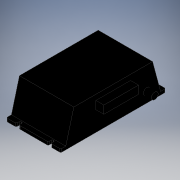
# Autodesk Inventor part: 12v_dc_to_dc
Saved by Autodesk Inventor 2017 (Build 210142000, 142)
## iProperties
Created: 2017-02-10
Part Number: 12v_dc_to_dc
Material: Generic
Document SubType Name: Modeling
Designer: michael
Density: 1 g/cm^3
Appearance: Default
Author: michael
Autodesk Inventor part; units mm, degrees
ref_plane "YZ Plane" through (0, 0, 0) normal (1, 0, 0) x (0, 1, 0)
ref_plane "XZ Plane" through (0, 0, 0) normal (0, 1, 0) x (-1, 0, 0)
ref_plane "XY Plane" through (0, 0, 0) normal (0, 0, 1) x (1, 0, 0)
sketch "Sketch1" plane through (0, 0, 0) normal (0, 1, 0) x (-1, 0, 0)
  line L0 (-51, 98.425) -> (51, 98.425)
  line L1 (51, 98.425) -> (51, -98.425)
  line L2 (51, -98.425) -> (-51, -98.425)
  line L3 (-51, -98.425) -> (-51, 98.425)
  line L4 (-51, 98.425) -> (51, -98.425) construction
  line L5 (51, 98.425) -> (-51, -98.425) construction
  point P0 (0, 0)
  dimension "d0" = 102
  dimension "d1" = 196.85
  constraints: 12 end point, 2 midpoint, 2 parallel, 1 horizontal, 1 perpendicular
  measures "d0" distance of L1.end L2.end
  measures "d1" distance of L0.end L1.end
extrude "Extrusion1" add sketch "Sketch1" along normal blind 6
sketch "Sketch2" plane through (0, 6, 0) normal (0, 1, 0) x (1, 0, 0)
  line L0 (51, -88.9) -> (-51, -88.9)
  line L1 (-51, -88.9) -> (-51, 88.9)
  line L2 (-51, 88.9) -> (51, 88.9)
  line L3 (51, 88.9) -> (51, -88.9)
  line L4 (51, -88.9) -> (-51, 88.9) construction
  line L5 (-51, -88.9) -> (51, 88.9) construction
  point P0 (0, 0)
  dimension "d4" = 102
  dimension "d5" = 177.8
  constraints: 12 end point, 2 midpoint, 2 parallel, 1 horizontal, 1 perpendicular
  measures "d4" distance of L1.end L2.end
  measures "d5" distance of L0.end L1.end
extrude "Extrusion2" add sketch "Sketch2" along normal blind 56
draft "FaceDraft1" angle 15 pull direction (0, 1, 0) faces at (17, 24.6667, 88.9) fixed edges at (0, 6, 88.9)
draft "FaceDraft2" angle 15 pull direction (0, 1, 0) faces at (-17, 24.6667, -88.9) fixed edges at (0, 6, -88.9)
sketch "Sketch3" plane through (0, 0, 0) normal (0, -1, 0) x (1, 0, 0)
  line L0 (32.4713, 98.425) -> (27.4713, 98.425)
  line L1 (27.4713, 98.425) -> (27.4713, 90.925)
  line L2 (27.4713, 90.925) -> (32.4713, 90.925)
  line L3 (32.4713, 90.925) -> (32.4713, 98.425)
  line L4 (32.4713, 98.425) -> (27.4713, 90.925) construction
  line L5 (27.4713, 98.425) -> (32.4713, 90.925) construction
  line L6 (51, -98.425) -> (51, 98.425) projected
  line L7 (-51, 98.425) -> (51, 98.425) projected
  line L8 (-27.4727, 90.925) -> (-32.4727, 90.925)
  line L9 (-32.4727, 90.925) -> (-32.4727, 98.425)
  line L10 (-32.4727, 98.425) -> (-27.4727, 98.425)
  line L11 (-27.4727, 98.425) -> (-27.4727, 90.925)
  line L12 (-27.4727, 90.925) -> (-32.4727, 98.425) construction
  line L13 (-32.4727, 90.925) -> (-27.4727, 98.425) construction
  line L14 (-51, 98.425) -> (-51, -98.425) projected
  line L15 (51, 0) -> (-51, 0)
  line L16 (-51, -73.8948) -> (-51, 73.8948) projected
  line L17 (32.4713, -98.425) -> (27.4713, -98.425)
  line L18 (27.4713, -98.425) -> (27.4713, -90.925)
  line L19 (27.4713, -90.925) -> (32.4713, -90.925)
  line L20 (32.4713, -90.925) -> (32.4713, -98.425)
  line L21 (-27.4727, -90.925) -> (-32.4727, -90.925)
  line L22 (-32.4727, -90.925) -> (-32.4727, -98.425)
  line L23 (-32.4727, -98.425) -> (-27.4727, -98.425)
  line L24 (-27.4727, -98.425) -> (-27.4727, -90.925)
  point P0 (0, 0)
  point P1 (29.9713, 94.675)
  point P2 (-29.9727, 94.675)
  point P3 (29.9713, -94.675)
  dimension "d10" = 5
  dimension "d11" = 7.5
  dimension "d12" = 21.0287
  dimension "d13" = 7.5
  dimension "d14" = 5
  dimension "d16" = 59.944
  dimension "d17" = 0
  constraints: 42 end point, 9 symmetric about line, 6 midpoint, 4 parallel, 2 horizontal, 2 perpendicular, 1 point on line
  measures "d10" distance of L2.end L1.end
  measures "d11" distance of L1.end L0.end
  measures "d12" distance from line of point (29.971, 94.675) L6
  measures "d13" distance between parallel lines of L8 L7
  measures "d14" distance between parallel lines of L9 L11
  measures "d16" distance of point (-29.973, 94.675) point (29.971, 94.675)
  measures "d17" distance between parallel lines of L7 L0
extrude "Extrusion3" cut sketch "Sketch3" against normal blind 56 contours L3 L2 L1 L0 | L11 L8 L9 L7 | L17 L18 L19 L20 | L24 L23 L22 L21
fillet "Fillet1" radius 2.159 20 edges at (27.4713, 3, 90.925) (32.4713, 3, 90.925) (32.4713, 3, 98.425) (27.4713, 3, 98.425) (-27.4727, 3, 90.925) (-32.4727, 3, 90.925) (-32.4727, 3, 98.425) (-27.4727, 3, 98.425) (-27.4727, 3, -98.425) (-27.4727, 3, -90.925) (-32.4727, 3, -90.925) (-32.4727, 3, -98.425) (27.4713, 3, -90.925) (27.4713, 3, -98.425) (32.4713, 3, -90.925) (32.4713, 3, -98.425) (51, 3, -98.425) (-51, 3, -98.425) (-51, 3, 98.425) (51, 3, 98.425)
sketch "Sketch4" plane through (51, 62, 73.8948) normal (1, 0, 0) x (0, 0, -1)
  line L0 (41.3948, -25) -> (106.3948, -25)
  line L1 (106.3948, -25) -> (106.3948, -10)
  line L2 (106.3948, -10) -> (41.3948, -10)
  line L3 (41.3948, -10) -> (41.3948, -25)
  line L4 (41.3948, -25) -> (106.3948, -10) construction
  line L5 (106.3948, -25) -> (41.3948, -10) construction
  line L6 (0, 0) -> (147.7897, 0) projected
  circle A0 centre (136.9784, -42.8226) radius 6.25
  point P0 (73.8948, -62)
  point P1 (73.8948, -17.5)
  dimension "d21" = 65
  dimension "d22" = 15
  dimension "d23" = 17.5
  dimension "d24" = 12.5
  constraints: 12 end point, 2 midpoint, 2 parallel, 1 centre point, 1 horizontal, 1 perpendicular
  measures "d21" distance of L2.end L1.end
  measures "d22" distance of L1.end L0.end
  measures "d23" distance from line of point (73.895, -17.5) L6
  measures "d24" diameter of A0
extrude "Extrusion4" add sketch "Sketch4" along normal blind 15
equation "\"d13\" = d11"
equation "\"d14\" = d10"
body "Solid1"
